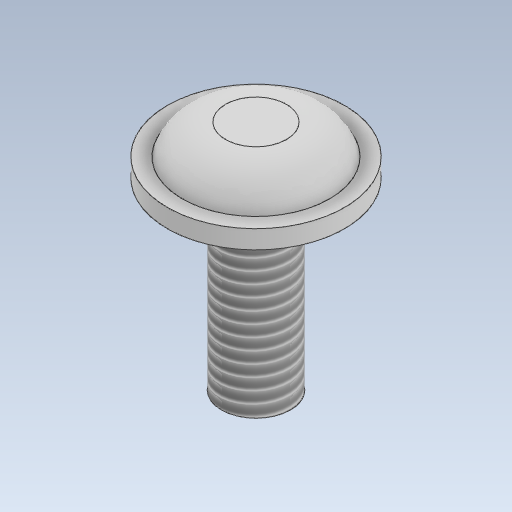
# Autodesk Inventor part: ClampHorn_Screw
Saved by Autodesk Inventor 2020 (Build 240168000, 168)
## iProperties
Created: 2021-08-24
Part Number: ClampHorn_Screw
Material: 一般
Document SubType Name: Modeling
Designer: naoki
Density: 1 g/cm^3
Appearance: 既定
Description: ネジ
Author: naoki
Autodesk Inventor part; units mm, degrees
ref_plane "YZ Plane" through (0, 0, 0) normal (1, 0, 0) x (0, 1, 0)
ref_plane "XZ Plane" through (0, 0, 0) normal (0, 1, 0) x (-1, 0, 0)
ref_plane "XY Plane" through (0, 0, 0) normal (0, 0, 1) x (1, 0, 0)
sketch "スケッチ1" plane through (0, 0, 0) normal (0, 1, 0) x (-1, 0, 0)
  circle A0 centre (0, 0) radius 3.85
  circle A1 centre (0, 0) radius 1.5
  circle A2 centre (0, 0) radius 3.2
  dimension "d0" = 7.7
  dimension "d1" = 3
  dimension "d6" = 6.4
  constraints: 3 centre point, 3 coincident
  measures "d0" diameter of A0
  measures "d1" diameter of A1
  measures "d6" diameter of A2
extrude "押し出し1" add sketch "スケッチ1" against normal blind 8 contours A1
extrude "押し出し2" add sketch "スケッチ1" along normal blind 0.8 contours A0 | A1 | A2
extrude "押し出し3" add sketch "スケッチ1" along normal blind 2.1 contours A1 | A2
fillet "フィレット1" radius 2 1 edges at (3.2, 2.1, 0)
thread "ねじ1" size "M3x0.5" class "6g" standard "ANSI Metric M Profile" full length
